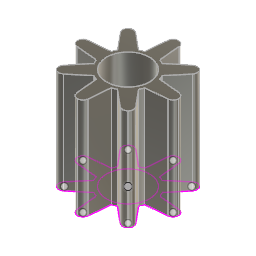
Small Head Gear (Autodesk Fusion 360 design; units mm, degrees)
Autodesk Fusion 360 part; units mm, degrees
note: some values were not read from the file. Set by a fixed rule: which sketch regions a step uses.
sketch "Small Head Gear" plane through (0, 0, 0) normal (0, 0, 1) x (1, 0, 0)
  circle A0 centre (0, 0) radius 1.0625
  arc A1 (-0.583, -1.1057) -> (-0.3696, -1.1941) centre (0, 0) ccw
  arc A2 (-1.1941, -0.3696) -> (-1.1057, -0.583) centre (0, 0) ccw
  arc A3 (-1.1057, 0.583) -> (-1.1941, 0.3696) centre (0, 0) ccw
  arc A4 (-0.3696, 1.1941) -> (-0.583, 1.1057) centre (0, 0) ccw
  arc A5 (0.583, 1.1057) -> (0.3696, 1.1941) centre (0, 0) ccw
  arc A6 (1.1941, 0.3696) -> (1.1057, 0.583) centre (0, 0) ccw
  arc A7 (0.3696, -1.1941) -> (0.583, -1.1057) centre (0, 0) ccw
  arc A8 (1.1057, -0.583) -> (1.1941, -0.3696) centre (0, 0) ccw
  line L0 (0, -2.5) -> (0.001, -2.5)
  line L1 (0, -2.5) -> (-0.001, -2.5)
  line L2 (1.7678, -1.7678) -> (1.7684, -1.7671)
  line L3 (1.7678, -1.7678) -> (1.7671, -1.7684)
  line L4 (1.7678, 1.7678) -> (1.7671, 1.7684)
  line L5 (1.7678, 1.7678) -> (1.7684, 1.7671)
  line L6 (0, 2.5) -> (-0.001, 2.5)
  line L7 (0, 2.5) -> (0.001, 2.5)
  line L8 (-1.7678, 1.7678) -> (-1.7684, 1.7671)
  line L9 (-1.7678, 1.7678) -> (-1.7671, 1.7684)
  line L10 (-2.5, 0) -> (-2.5, -0.001)
  line L11 (-2.5, 0) -> (-2.5, 0.001)
  line L12 (-1.7678, -1.7678) -> (-1.7671, -1.7684)
  line L13 (-1.7678, -1.7678) -> (-1.7684, -1.7671)
  line L14 (-0.3696, -1.1941) -> (-0.2729, -2.2501)
  line L15 (0.2729, -2.2501) -> (0.3696, -1.1941)
  line L16 (0.583, -1.1057) -> (1.3981, -1.784)
  line L17 (1.784, -1.3981) -> (1.1057, -0.583)
  line L18 (1.1941, -0.3696) -> (2.2501, -0.2729)
  line L19 (2.2501, 0.2729) -> (1.1941, 0.3696)
  line L20 (1.1057, 0.583) -> (1.784, 1.3981)
  line L21 (1.3981, 1.784) -> (0.583, 1.1057)
  line L22 (0.3696, 1.1941) -> (0.2729, 2.2501)
  line L23 (-0.2729, 2.2501) -> (-0.3696, 1.1941)
  line L24 (-0.583, 1.1057) -> (-1.3981, 1.784)
  line L25 (-1.784, 1.3981) -> (-1.1057, 0.583)
  line L26 (-1.1941, 0.3696) -> (-2.2501, 0.2729)
  line L27 (-2.2501, -0.2729) -> (-1.1941, -0.3696)
  line L28 (-1.1057, -0.583) -> (-1.784, -1.3981)
  line L29 (-1.3981, -1.784) -> (-0.583, -1.1057)
  line L30 (2.5, -0.001) -> (2.5, 0.001)
  arc A9 (-0.2729, -2.2501) -> (0.001, -2.5) centre (0.001, -2.225) ccw
  arc A10 (-0.001, -2.5) -> (0.2729, -2.2501) centre (-0.001, -2.225) ccw
  arc A11 (1.3981, -1.784) -> (1.7684, -1.7671) centre (1.574, -1.5726) ccw
  arc A12 (1.7671, -1.7684) -> (1.784, -1.3981) centre (1.5726, -1.574) ccw
  arc A13 (2.2501, -0.2729) -> (2.5, 0.001) centre (2.225, 0.001) ccw
  arc A14 (2.5, -0.001) -> (2.2501, 0.2729) centre (2.225, -0.001) ccw
  arc A15 (1.784, 1.3981) -> (1.7671, 1.7684) centre (1.5726, 1.574) ccw
  arc A16 (1.7684, 1.7671) -> (1.3981, 1.784) centre (1.574, 1.5726) ccw
  arc A17 (0.2729, 2.2501) -> (-0.001, 2.5) centre (-0.001, 2.225) ccw
  arc A18 (0.001, 2.5) -> (-0.2729, 2.2501) centre (0.001, 2.225) ccw
  arc A19 (-1.3981, 1.784) -> (-1.7684, 1.7671) centre (-1.574, 1.5726) ccw
  arc A20 (-1.7671, 1.7684) -> (-1.784, 1.3981) centre (-1.5726, 1.574) ccw
  arc A21 (-2.2501, 0.2729) -> (-2.5, -0.001) centre (-2.225, -0.001) ccw
  arc A22 (-2.5, 0.001) -> (-2.2501, -0.2729) centre (-2.225, 0.001) ccw
  arc A23 (-1.7684, -1.7671) -> (-1.3981, -1.784) centre (-1.574, -1.5726) ccw
  arc A24 (-1.784, -1.3981) -> (-1.7671, -1.7684) centre (-1.5726, -1.574) ccw
  constraint coincident A0.centre A1.centre
  constraint concentric A1 A7
  constraint concentric A2 A7
  constraint concentric A3 A7
  constraint coincident A4.start A7
  constraint concentric A4 A7
  constraint concentric A5 A7
  constraint concentric A6 A7
  constraint concentric A7 A8
  constraint vertical L30
  constraint tangent L0 A9
  constraint tangent L14 A9
  constraint tangent L1 A10
  constraint tangent L15 A10
  constraint tangent L2 A11
  constraint tangent L16 A11
  constraint tangent L3 A12
  constraint tangent L17 A12
  constraint tangent L18 A13
  constraint tangent L30 A13
  constraint tangent L19 A14
  constraint tangent L30 A14
  constraint tangent L4 A15
  constraint tangent L20 A15
  constraint tangent L5 A16
  constraint tangent L21 A16
  constraint tangent L22 A17
  constraint tangent L6 A17
  constraint tangent L7 A18
  constraint tangent L23 A18
  constraint tangent L8 A19
  constraint tangent L24 A19
  constraint tangent L9 A20
  constraint tangent L25 A20
  constraint tangent L26 A21
  constraint tangent L10 A21
  constraint tangent L11 A22
  constraint tangent L27 A22
  constraint tangent L13 A23
  constraint tangent L29 A23
  constraint tangent L12 A24
  constraint tangent L28 A24
extrude "Extrude1" add sketch "Small Head Gear" along normal blind 5
named bodies: "Small Head Gear"
